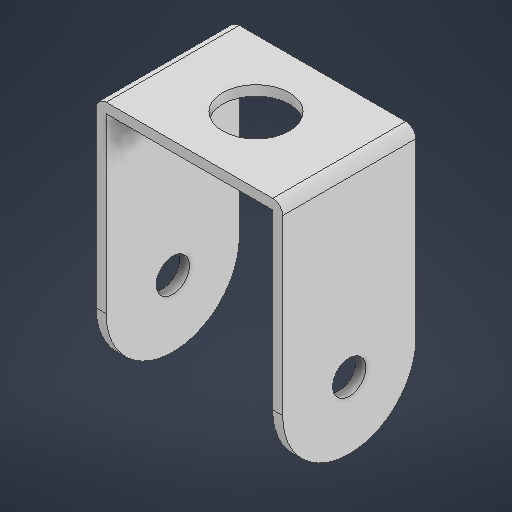
# Autodesk Inventor part: Part1dia7demaio
Saved by Autodesk Inventor 2026 (Build 300175050, 175E)
## iProperties
Created: 2026-05-07
Part Number: Part1dia7demaio
Material: Generic
Document SubType Name: Modeling
Designer: Administrator
Density: 1 g/cm^3
Appearance: Default
Author: Administrator
Autodesk Inventor part; units mm, degrees
ref_plane "YZ Plane" through (0, 0, 0) normal (1, 0, 0) x (0, 1, 0)
ref_plane "XZ Plane" through (0, 0, 0) normal (0, 1, 0) x (-1, 0, 0)
ref_plane "XY Plane" through (0, 0, 0) normal (0, 0, 1) x (1, 0, 0)
sketch "Sketch1" plane through (0, 0, 0) normal (0, 0, 1) x (1, 0, 0)
  line L0 (0, 0) -> (3, 0)
  line L1 (3, 0) -> (3, 72)
  line L2 (3, 72) -> (53, 72)
  line L3 (53, 72) -> (53, 0)
  line L4 (53, 0) -> (56, 0)
  line L5 (56, 0) -> (56, 75)
  line L6 (56, 75) -> (0, 75)
  line L7 (0, 75) -> (0, 0)
  dimension "d0" = 75
  dimension "d1" = 50
  dimension "d2" = 3
  dimension "d3" = 3
  dimension "d4" = 3
  constraints: 16 end point, 6 perpendicular, 2 point on line, 1 horizontal
  measures "d0" distance of L6.end L0.start
  measures "d1" distance between parallel lines of L3 L1
  measures "d2" distance between parallel lines of L2 L6
  measures "d3" distance between parallel lines of L7 L1
  measures "d4" distance between parallel lines of L5 L3
extrude "Extrusion1" add sketch "Sketch1" along normal mid plane 40
fillet "Fillet1" radius 3 1 edges at (56, 75, 0)
fillet "Fillet2" radius 3 1 edges at (0, 75, 0)
fillet "Fillet3" radius 20 1 edges at (54.5, 0, 20)
fillet "Fillet4" radius 20 1 edges at (1.5, 0, 20)
fillet "Fillet5" radius 20 1 edges at (54.5, 0, -20)
fillet "Fillet6" radius 20 1 edges at (1.5, 0, -20)
sketch "Sketch2" plane through (56, 72, 20) normal (1, 0, 0) x (0, 0, -1)
  arc A0 (0, -52) -> (40, -52) centre (20, -52) ccw projected
  circle A1 centre (20, -52) radius 5
  point P0 (20, -72)
  dimension "d13" = 10
  constraints: 1 centre point, 1 coincident
  measures "d13" diameter of A1
extrude "Extrusion2" cut sketch "Sketch2" against normal through all
sketch "Sketch3" plane through (53, 75, 20) normal (0, 1, 0) x (1, 0, 0)
  line L0 (-53, 20) -> (3, 20) construction
  line L1 (3, 25) -> (3, 15) projected
  circle A0 centre (-25, 20) radius 10
  dimension "d16" = 20
  constraints: 2 end point, 2 midpoint, 1 centre point
  measures "d16" diameter of A0
extrude "Extrusion3" cut sketch "Sketch3" against normal blind 10
body "Solid1"
